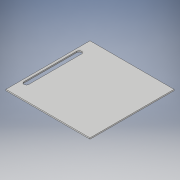
# Autodesk Inventor part: Top Plate
Saved by Autodesk Inventor 2019 (Build 230136000, 136)
## iProperties
Created: 2019-03-05
Part Number: Top Plate
Material: Nylon 6/6
Document SubType Name: Modeling
Designer: Delta
Density: 1.13 g/cm^3
Appearance: Default
Mass: 1417.74 g
Surface Area: 4064.51 cm^2
Volume: 1254.63 cm^3
Author: Delta
Autodesk Inventor part; units mm, degrees
ref_plane "YZ Plane" through (0, 0, 0) normal (1, 0, 0) x (0, 1, 0)
ref_plane "XZ Plane" through (0, 0, 0) normal (0, 1, 0) x (-1, 0, 0)
ref_plane "XY Plane" through (0, 0, 0) normal (0, 0, 1) x (1, 0, 0)
sketch "Sketch1" plane through (0, 0, 0) normal (0, 1, 0) x (-1, 0, 0)
  line L0 (0, 0) -> (444.5, 0)
  line L1 (444.5, 0) -> (444.5, -444.5)
  line L2 (444.5, -444.5) -> (0, -444.5)
  line L3 (0, -444.5) -> (0, 0)
  dimension "d0" = 444.5
  dimension "d1" = 444.5
  constraints: 8 end point, 2 parallel, 1 horizontal, 1 perpendicular
  measures "d0" distance of L1.end L2.end
  measures "d1" distance of L0.end L1.end
extrude "Extrusion1" add sketch "Sketch1" along normal blind 6.35
sketch "Sketch2" plane through (0, 6.35, 0) normal (0, 1, 0) x (1, 0, 0)
  line L0 (-444.5, 0) -> (0, 0) projected
  line L1 (-444.5, 444.5) -> (-444.5, 0) projected
  line L2 (-419.1, 374.65) -> (-419.1, 69.85) construction
  line L3 (-431.8, 361.95) -> (-431.8, 82.55)
  line L4 (-406.4, 82.55) -> (-406.4, 361.95)
  arc A0 (-406.4, 361.95) -> (-431.8, 361.95) centre (-419.1, 361.95) ccw
  arc A1 (-431.8, 82.55) -> (-406.4, 82.55) centre (-419.1, 82.55) ccw
  line L5 (0, 444.5) -> (-444.5, 444.5) projected
  point P0 (-419.1, 222.25)
  dimension "d8" = 444.5
  dimension "d12" = 25.4
  dimension "d13" = 12.7
  dimension "d14" = 304.8
  dimension "d15" = 69.85
  constraints: 8 end point, 6 point on circle, 4 tangent, 2 centre point, 2 point on line, 1 midpoint, 1 parallel, 1 vertical
  measures "d8" distance of L0.start L0.end
  measures "d12" diameter of A1
  measures "d13" distance between parallel lines of L1 L3
  measures "d14" distance of L2.end L2.start
  measures "d15" distance from line of L5 L2.start
extrude "Extrusion3" cut sketch "Sketch2" against normal through all
equation "\"d15\" = -0.5 * d14 + 0.5 * d8"
body "Solid1"
